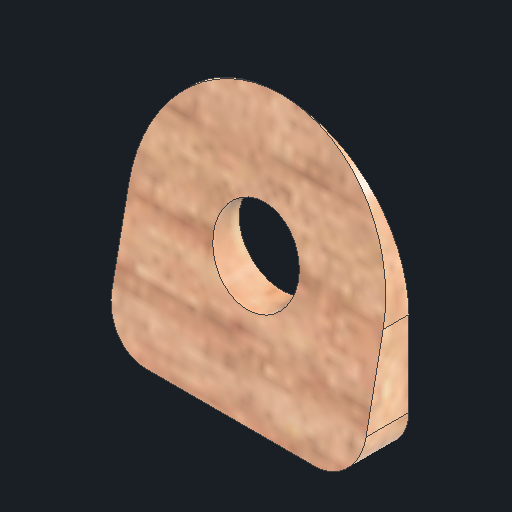
# Autodesk Inventor part: TRI_SPACER_TOP_TREBUCHET
Saved by Autodesk Inventor 2026.2 (Build 302298010, 298A)
## iProperties
Created: 2026-02-19
Part Number: TRI_SPACER_TOP_TREBUCHET
Material: Wood (Birch)
Document SubType Name: Modeling
Designer: 4aida
Density: 0.55 g/cm^3
Appearance: Birch - Natural Polished
Mass: 2.65233 g
Surface Area: 30.3209 cm^2
Volume: 4.82241 cm^3
Author: 4aida
Autodesk Inventor part; units mm, degrees
ref_plane "YZ Plane" through (0, 0, 0) normal (1, 0, 0) x (0, 1, 0)
ref_plane "XZ Plane" through (0, 0, 0) normal (0, 1, 0) x (-1, 0, 0)
ref_plane "XY Plane" through (0, 0, 0) normal (0, 0, 1) x (1, 0, 0)
sketch "Sketch1" plane through (0, 0, 0) normal (1, 0, 0) x (0, 1, 0)
  line L0 (0, 0) -> (-38.1, 7.674)
  line L1 (-38.1, 7.674) -> (-38.1, 0)
  line L2 (-38.1, 0) -> (0, 0)
  dimension "d0" = 38.1
  dimension "d1" = 11.388
  constraints: 6 end point, 1 perpendicular, 1 vertical
  measures "d0" distance of L0.start L1.end
  measures "d1" angle of L2 L0
extrude "Extrusion1" add sketch "Sketch1" along normal blind 38.1
sketch "Sketch2" plane through (0, -38.1, 0) normal (0, 0, -1) x (-1, 0, 0)
  circle A0 centre (-19.05, 19.05) radius 19.05
  line L0 (0, 38.1) -> (-38.1, 38.1) projected
  line L1 (0, 0) -> (0, 38.1) projected
  line L2 (-38.1, 0) -> (-38.1, 38.1) projected
  circle A1 centre (-19.05, 19.05) radius 6.35
  point P0 (-38.1, 19.05)
  point P1 (-19.05, 38.1)
  point P2 (0, 19.05)
  dimension "d4" = 12.7
  constraints: 3 tangent, 2 centre point, 1 coincident
  measures "d4" diameter of A1
extrude "Extrusion2" cut sketch "Sketch2" against normal through all contours A0 L0 L1 | A0 L2 L0 | A1
fillet "Fillet1" radius 6.35 2 edges at (38.1, -38.1, 3.837) (0, -38.1, 3.837)
body "Solid1"
